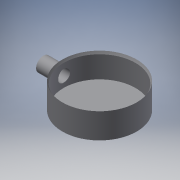
# Autodesk Inventor part: low_profile_noiseAttachment
Saved by Autodesk Inventor 2016 (Build 200138000, 138)
## iProperties
Created: 2012-05-12
Part Number: low_profile_noiseAttachment
Material: Generic
Document SubType Name: Modeling
Designer: charvey
Density: 1 g/cm^3
Appearance: Default
Author: charvey
Autodesk Inventor part; units mm, degrees
ref_plane "YZ Plane" through (0, 0, 0) normal (1, 0, 0) x (0, 1, 0)
ref_plane "XZ Plane" through (0, 0, 0) normal (0, 1, 0) x (-1, 0, 0)
ref_plane "XY Plane" through (0, 0, 0) normal (0, 0, 1) x (1, 0, 0)
sketch "Sketch1" plane through (0, 0, 0) normal (0, 0, 1) x (1, 0, 0)
  line L0 (87.9882, 31.75) -> (89.8166, 31.75)
  line L1 (0, 0) -> (0, -1.5875)
  line L2 (0, -30.1625) -> (95.25, -30.1625)
  line L3 (0, -30.1625) -> (0, -26.9875)
  line L4 (95.25, -30.1625) -> (95.25, 34.519)
  line L5 (0, -26.9875) -> (92.075, -26.9875)
  line L6 (92.075, -26.9875) -> (92.075, 28.6057)
  arc A0 (92.075, 28.6057) -> (95.25, 34.519) centre (0, 81.8521) ccw
  dimension "d11" = 31.75
  dimension "d52" = 95.25
  dimension "d53" = 3.175
  dimension "d55" = 3.175
  dimension "d56" = 106.3625
  constraints: 14 end point, 5 perpendicular, 2 point on circle, 1 centre point, 1 parallel
  measures "d11" vertical distance of L1.start L0.start
  measures "d52" distance of L2.end L2.start
  measures "d53" distance of L2.start L3.end
  measures "d55" horizontal distance of L2.end L5.end
  measures "d56" radius of A0
revolve "Revolution4" add sketch "Sketch1" angle 360 about axis through (0, -30.1625, 0) along (0, 1, 0)
sketch "Sketch15" plane through (0, 0, 0) normal (0, 1, 0) x (-1, 0, 0)
  line L0 (144.2529, 0) -> (144.2529, -18.415)
  circle A0 centre (0, 0) radius 95.25 projected
  line L1 (144.2529, -18.415) -> (93.4529, -18.415)
  line L2 (144.2529, 0) -> (141.0779, 0)
  line L3 (141.0779, 0) -> (141.0779, -15.24)
  line L4 (141.0779, -15.24) -> (94.0229, -15.24)
  point P0 (0, 0)
  dimension "d58" = 3.175
  dimension "d59" = 15.24
  dimension "d60" = 3.175
  dimension "d61" = 50.8
  constraints: 10 end point, 3 perpendicular, 2 point on circle, 1 horizontal alignment, 1 parallel, 1 vertical
  measures "d58" distance between parallel lines of L1 L4
  measures "d59" distance of L3.end L2.end
  measures "d60" distance between parallel lines of L3 L0
  measures "d61" distance of L0.end L1.end
revolve "Revolution5" add sketch "Sketch15" angle 360 about axis through (-144.2529, 0, 0) along (1, 0, 0) contours L0 L1 A0 L4 L3 L2
sketch "Sketch17" plane through (-144.2529, 0, 0) normal (-1, 0, 0) x (0, 0, 1)
  circle A0 centre (0, 0) radius 18.415 projected
  constraints: 1 coincident
hole "Hole5" at (-144.2529, 0, 0) direction (1, 0, 0) diameter 30.48 depth 127 tip angle 118
sketch "Sketch18" plane through (-144.2529, 0, 0) normal (-1, 0, 0) x (0, 0, 1)
  point P0 (0, 0)
body "Solid3"
